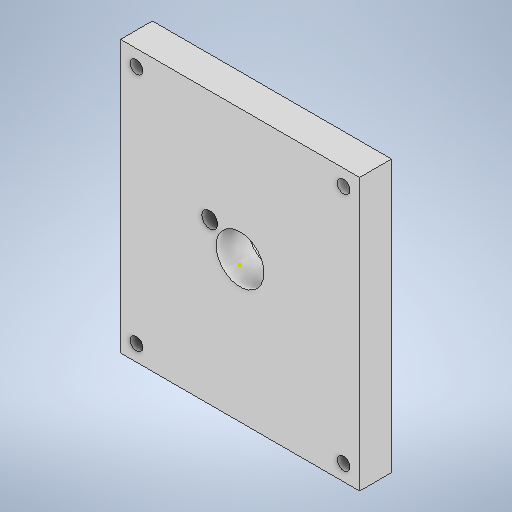
# Autodesk Inventor part: Rb PEEK - Corto con ventana
Saved by Autodesk Inventor 2025.3 (Build 293356000, 356)
## iProperties
Created: 2025-05-09
Part Number: Rb PEEK - Corto con ventana
Material: Generic
Document SubType Name: Modeling
Designer: E. Moreno
Density: 1 g/cm^3
Appearance: Default
Author: E. Moreno
Title: Rb PEEK - Corto con ventana
Autodesk Inventor part; units mm, degrees
ref_plane "YZ Plane" through (0, 0, 0) normal (1, 0, 0) x (0, 1, 0)
ref_plane "XZ Plane" through (0, 0, 0) normal (0, 1, 0) x (-1, 0, 0)
ref_plane "XY Plane" through (0, 0, 0) normal (0, 0, 1) x (1, 0, 0)
sketch "Sketch1" plane through (0, 0, 0) normal (0, 0, 1) x (1, 0, 0)
  line L0 (-37.5, -42.6) -> (37.5, -42.6)
  line L1 (37.5, -42.6) -> (37.5, 42.6)
  line L2 (37.5, 42.6) -> (-37.5, 42.6)
  line L3 (-37.5, 42.6) -> (-37.5, -42.6)
  line L4 (-37.5, -42.6) -> (37.5, 42.6) construction
  line L5 (37.5, -42.6) -> (-37.5, 42.6) construction
  point P0 (0, 0)
  dimension "d0" = 75
  dimension "d1" = 85.2
  constraints: 12 end point, 2 midpoint, 2 parallel, 1 horizontal, 1 perpendicular
  measures "d0" distance of L2.end L1.end
  measures "d1" distance of L1.end L0.end
extrude "Extrusion1" add sketch "Sketch1" along normal blind 10
sketch "Sketch4" plane through (0, 0, 10) normal (0, 0, 1) x (1, 0, 0)
  point P0 (0, 0)
sketch "Sketch5" plane through (0, 0, 10) normal (0, 0, 1) x (1, 0, 0)
  line L0 (-37.5, -42.6) -> (37.5, -42.6) projected
  line L1 (0, -42.6) -> (0, 1.6)
  circle A0 centre (0, 1.6) radius 7.5
  line L2 (0, 1.6) -> (13, 1.6)
  point P0 (0, 0)
  dimension "d21" = 44.2
  dimension "d22" = 15
  constraints: 4 end point, 1 centre point, 1 coincident, 1 horizontal, 1 midpoint, 1 vertical
  measures "d21" distance of L1.start L1.end
  measures "d22" diameter of A0
extrude "Extrusion6" cut sketch "Sketch5" against normal blind 10
sketch "Sketch6" plane through (0, 0, 10) normal (0, 0, 1) x (1, 0, 0)
  circle A0 centre (13, 6.6) radius 3.75 projected
sketch "Boceto7" plane through (0, 0, 0) normal (0, 0, -1) x (-1, 0, 0)
  circle A0 centre (0, 1.6) radius 3.9163
  circle A1 centre (0, 1.6) radius 7.5 projected
  line L0 (0, 1.6) -> (9.5, 1.6)
  line L1 (9.5, 1.6) -> (9.5, 7.6)
  circle A2 centre (9.5, 7.6) radius 2.5
  point P0 (0, 0)
  dimension "d38" = 9.5
  dimension "d39" = 6
  dimension "d40" = 5
  constraints: 4 end point, 2 centre point, 1 coincident, 1 concentric, 1 horizontal, 1 perpendicular
  measures "d38" distance of L0.start L0.end
  measures "d39" distance of L0.end L1.end
  measures "d40" diameter of A2
extrude "Extrusión7" cut sketch "Boceto7" against normal blind 10 contours A2
sketch "Boceto8" plane through (0, 0, 10) normal (0, 0, 1) x (1, 0, 0)
  circle A0 centre (-9.5, 7.6) radius 2.5 projected
sketch "Boceto9" plane through (0, 0, 0) normal (0, 0, -1) x (-1, 0, 0)
  circle A0 centre (9.5, 7.6) radius 2.5 projected
sketch "Boceto10" plane through (0, 0, 10) normal (0, 0, 1) x (1, 0, 0)
  circle A0 centre (-9.5, 7.6) radius 2.5 projected
sketch "Boceto11" plane through (0, 0, 0) normal (0, 0, -1) x (-1, 0, 0)
  circle A0 centre (9.5, 7.6) radius 2.5 projected
sketch "Sketch12" plane through (0, 0, 10) normal (0, 0, 1) x (1, 0, 0)
  point P0 (0, 0)
sketch "Sketch13" plane through (0, 0, 10) normal (0, 0, 1) x (1, 0, 0)
  line L0 (37.5, -42.6) -> (37.5, 42.6) projected
  line L1 (37.5, -42.6) -> (32.5, -42.6)
  line L2 (-37.5, -42.6) -> (37.5, -42.6) projected
  line L3 (32.5, -42.6) -> (32.5, -37.6)
  circle A0 centre (32.5, -37.6) radius 2
  circle A1 centre (32.5, -37.6) radius 3.61
  line L4 (0, 0) -> (0, -42.6)
  line L5 (-37.5, 42.6) -> (-37.5, -42.6) projected
  line L6 (-37.5, 0) -> (37.5, 0)
  line L7 (-32.5, -42.6) -> (-32.5, -37.6)
  circle A2 centre (-32.5, -37.6) radius 2
  circle A3 centre (-32.5, -37.6) radius 3.61
  line L8 (37.5, 42.6) -> (32.5, 42.6)
  line L9 (-37.5, 42.6) -> (37.5, 42.6)
  line L10 (32.5, 42.6) -> (32.5, 37.6)
  circle A4 centre (32.5, 37.6) radius 2
  circle A5 centre (32.5, 37.6) radius 3.61
  line L11 (-32.5, 42.6) -> (-32.5, 37.6)
  circle A6 centre (-32.5, 37.6) radius 2
  circle A7 centre (-32.5, 37.6) radius 3.61
  point P0 (0, 42.6)
  dimension "d43" = 5
  dimension "d44" = 5
  dimension "d45" = 4
  dimension "d46" = 7.22
  constraints: 18 end point, 13 symmetric about line, 8 centre point, 8 coincident, 3 midpoint, 2 point on line, 1 perpendicular, 6 other
  measures "d43" distance of L0.start L1.end
  measures "d44" distance of L1.end L3.end
  measures "d45" diameter of A0
  measures "d46" diameter of A1
extrude "Extrusion8" cut sketch "Sketch13" against normal blind 10 contours A0 | A2 | A4 | A6
sketch "Sketch15" plane through (0, 0, 0) normal (0, 0, -1) x (-1, 0, 0)
  circle A0 centre (32.5, 37.6) radius 2 projected
  circle A1 centre (32.5, 37.6) radius 3.61
  line L0 (-37.5, 42.6) -> (37.5, 42.6) projected
  line L1 (0, 42.6) -> (0, 0)
  line L2 (-37.5, -42.6) -> (-37.5, 42.6) projected
  line L3 (-37.5, 0) -> (37.5, 0)
  circle A2 centre (-32.5, 37.6) radius 2
  circle A3 centre (-32.5, 37.6) radius 3.61
  circle A4 centre (32.5, -37.6) radius 2
  circle A5 centre (32.5, -37.6) radius 3.61
  circle A6 centre (-32.5, -37.6) radius 2
  circle A7 centre (-32.5, -37.6) radius 3.61
  point P0 (0, -42.6)
  dimension "d52" = 7.22
  constraints: 7 centre point, 7 symmetric about line, 4 coincident, 4 end point, 2 midpoint, 1 horizontal, 1 vertical, 6 other
  measures "d52" diameter of A1
extrude "Extrusion10" cut sketch "Sketch15" against normal blind 4.5 contours A0 | A1 | A3 | A4 | A5 | A6 | A7
body "Solid1"
